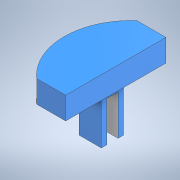
# Autodesk Inventor part: holder_for_wire
Saved by Autodesk Inventor 2022 (Build 260153000, 153)
## iProperties
Created: 2021-10-11
Part Number: holder_for_wire
Material: Generic
Document SubType Name: Modeling
Designer: Nikita
Density: 1 g/cm^3
Appearance: Default
Author: Nikita
Autodesk Inventor part; units mm, degrees
ref_plane "YZ Plane" through (0, 0, 0) normal (1, 0, 0) x (0, 1, 0)
ref_plane "XZ Plane" through (0, 0, 0) normal (0, 1, 0) x (-1, 0, 0)
ref_plane "XY Plane" through (0, 0, 0) normal (0, 0, 1) x (1, 0, 0)
sketch "Sketch1" plane through (0, 0, 0) normal (0, 1, 0) x (-1, 0, 0)
  line L0 (-5, 5) -> (5, 5) construction
  line L1 (5, 5) -> (5, -5) construction
  line L2 (5, -5) -> (-5, -5) construction
  line L3 (-5, -5) -> (-5, 5) construction
  line L4 (-5, 5) -> (5, -5) construction
  line L5 (5, 5) -> (-5, -5) construction
  line L6 (6.5, 22.5) -> (-6.5, 22.5)
  line L7 (-6.5, 22.5) -> (-6.5, -22.5)
  line L8 (-6.5, -22.5) -> (6.5, -22.5)
  line L9 (6.5, 22.5) -> (-6.5, -22.5) construction
  line L10 (-6.5, 22.5) -> (6.5, -22.5) construction
  arc A0 (6.5, -22.5) -> (6.5, 22.5) centre (-13.3431, 0) ccw
  point P0 (0, 0)
  dimension "d0" = 10
  dimension "d1" = 10
  dimension "d2" = 13
  dimension "d3" = 45
  dimension "d4" = 30
  constraints: 22 end point, 4 midpoint, 3 parallel, 2 horizontal, 2 perpendicular, 2 point on circle, 1 centre point
  measures "d0" distance of L1.end L2.end
  measures "d1" distance of L0.end L1.end
  measures "d2" distance of L8.end L7.end
  measures "d3" distance of L6.end L7.end
  measures "d4" radius of A0
extrude "Extrusion1" add sketch "Sketch1" along normal blind 10
sketch "Sketch2" plane through (0, 0, 0) normal (0, -1, 0) x (1, 0, 0)
  line L0 (-5, 5) -> (5, 5)
  line L1 (5, 5) -> (5, -5)
  line L2 (5, -5) -> (-5, -5)
  line L3 (-5, -5) -> (-5, 5)
  line L4 (-5, 5) -> (5, -5) construction
  line L5 (5, 5) -> (-5, -5) construction
  point P0 (0, 0)
  dimension "d7" = 10
  dimension "d8" = 10
  constraints: 12 end point, 2 midpoint, 2 parallel, 1 horizontal, 1 perpendicular
  measures "d7" distance of L1.end L2.end
  measures "d8" distance of L0.end L1.end
extrude "Extrusion2" add sketch "Sketch2" along normal blind 20
sketch "Sketch4" plane through (0, -20, 0) normal (0, -1, 0) x (1, 0, 0)
  line L0 (5, 5) -> (5, -5) projected
  line L1 (-5, 2.5) -> (5, 2.5)
  line L2 (5, 2.5) -> (5, -2.5)
  line L3 (5, -2.5) -> (-5, -2.5)
  line L4 (-5, -2.5) -> (-5, 2.5)
  line L5 (-5, 2.5) -> (5, -2.5) construction
  line L6 (5, 2.5) -> (-5, -2.5) construction
  line L7 (5, 5) -> (-5, 5) projected
  line L8 (-5, 5) -> (-5, -5) projected
  point P0 (0, 0)
  point P1 (5, 0)
  dimension "d11" = 5
  dimension "d14" = 10
  constraints: 12 end point, 3 midpoint, 2 parallel, 1 horizontal, 1 perpendicular
  measures "d11" distance of L1.end L2.end
  measures "d14" distance of L2.end L3.end
extrude "Extrusion3" cut sketch "Sketch4" against normal blind 18 contours L0 L3 L4 L1
body "Solid1"
